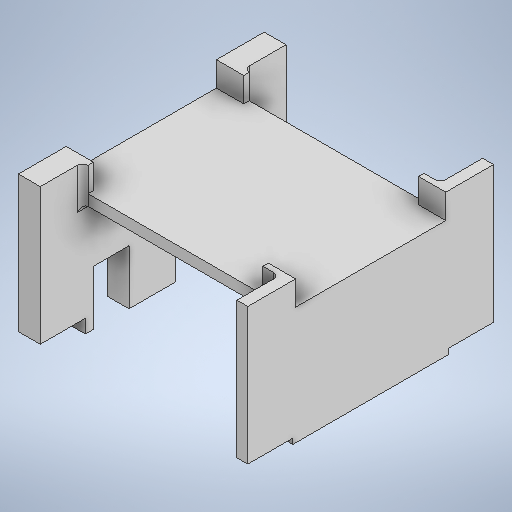
# Autodesk Inventor part: Breadboard_insert
Saved by Autodesk Inventor 2025.2 (Build 292293000, 293)
## iProperties
Created: 2025-09-19
Part Number: Breadboard_insert
Material: Generic
Document SubType Name: Modeling
Designer: TSO
Density: 1 g/cm^3
Appearance: Default
Author: TSO
Autodesk Inventor part; units mm, degrees
ref_plane "YZ Plane" through (0, 0, 0) normal (1, 0, 0) x (0, 1, 0)
ref_plane "XZ Plane" through (0, 0, 0) normal (0, 1, 0) x (-1, 0, 0)
ref_plane "XY Plane" through (0, 0, 0) normal (0, 0, 1) x (1, 0, 0)
sketch "Sketch1" plane through (0, 0, 0) normal (0, 1, 0) x (-1, 0, 0)
  line L0 (0, 0) -> (84, 0)
  line L1 (84, 0) -> (84, -90)
  line L2 (84, -90) -> (0, -90)
  line L3 (0, -90) -> (0, 0)
  line L4 (84, 0) -> (76, 0)
  line L5 (76, 0) -> (4, 0)
  line L6 (4, 0) -> (4, -15.5)
  line L7 (4, -15.5) -> (76, -15.5)
  line L8 (76, -15.5) -> (76, 0)
  line L9 (84, -45) -> (0, -45) construction
  line L10 (4, -90) -> (4, -74.5)
  line L11 (4, -74.5) -> (76, -74.5)
  line L12 (76, -74.5) -> (76, -90)
  point P0 (4, 0)
  point P1 (4, -90)
  dimension "d0" = 84
  dimension "d1" = 90
  dimension "d4" = 8
  dimension "d5" = 72
  dimension "d6" = 15.5
  constraints: 26 end point, 4 parallel, 4 symmetric about line, 2 horizontal, 2 midpoint, 2 perpendicular, 1 point on line
  measures "d0" distance of L1.end L2.end
  measures "d1" distance of L0.end L1.end
  measures "d4" distance of L0.end L4.end
  measures "d5" distance of L7.end L6.end
  measures "d6" distance of L6.end L5.end
extrude "Extrusion1" add sketch "Sketch1" along normal blind 4 contours L0 L6 L7 L8 L1 L2 L12 L11 L10 L3
sketch "Sketch2" plane through (0, 0, 0) normal (0, -1, 0) x (1, 0, 0)
  line L0 (-84, -90) -> (-84, 0) projected
  line L1 (-76, 0) -> (-76, -15.5) projected
  line L2 (-84, -90) -> (-76, -90)
  line L3 (-76, -90) -> (-76, 0)
  line L4 (-76, 0) -> (-84, 0)
  line L5 (-84, 0) -> (-84, -90)
  line L6 (0, -90) -> (0, 0)
  line L7 (0, 0) -> (0, -90) projected
  line L8 (-4, 0) -> (0, 0) projected
  line L9 (0, -90) -> (-4, -90)
  line L10 (-4, -90) -> (-4, 0)
  line L11 (-4, 0) -> (0, 0)
  line L12 (0, 0) -> (0, -90)
  dimension "d12" = 4
  constraints: 18 end point, 4 parallel, 2 horizontal, 2 perpendicular, 1 point on line
  measures "d12" distance of L10.end L11.end
extrude "Extrusion2" add sketch "Sketch2" along normal blind 37
sketch "Sketch3" plane through (0, -37, 0) normal (0, -1, 0) x (1, 0, 0)
  line L0 (-76, -74.5) -> (-76, -90) projected
  line L1 (-76, -74.5) -> (-76, -73.5)
  line L2 (-76, -15.5) -> (-76, -74.5) projected
  line L3 (-76, -73.5) -> (-84, -73.5)
  line L4 (-84, -73.5) -> (-84, -16.5)
  line L5 (-84, -16.5) -> (-76, -16.5)
  line L6 (-76, -16.5) -> (-76, -73.5)
  point P0 (0, 0)
  dimension "d17" = 1
  dimension "d18" = 8
  dimension "d19" = 57
  constraints: 10 end point, 2 parallel, 1 horizontal, 1 perpendicular, 1 point on line
  measures "d17" distance of L0.start L1.end
  measures "d18" distance of L4.end L5.end
  measures "d19" distance of L3.end L4.end
extrude "Extrusion3" add sketch "Sketch3" along normal blind 5
sketch "Sketch5" plane through (0, -37, 0) normal (0, -1, 0) x (1, 0, 0)
  line L0 (-4, -74.5) -> (-4, -73.5)
  line L1 (-4, -73.5) -> (-4, -73.5) construction
  line L2 (-4, 0) -> (-4, -90) projected
  line L3 (-4, -73.5) -> (0, -73.5)
  line L4 (0, -73.5) -> (0, -16.5)
  line L5 (0, -16.5) -> (-4, -16.5)
  line L6 (-4, -16.5) -> (-4, -73.5)
  point P0 (0, 0)
  dimension "d20" = 1
  dimension "d21" = 4
  dimension "d22" = 57
  constraints: 12 end point, 2 parallel, 2 perpendicular, 1 horizontal, 1 point on line, 1 vertical
  measures "d20" distance of L0.start L0.end
  measures "d21" distance of L5.end L4.end
  measures "d22" distance of L4.end L3.end
extrude "Extrusion4" add sketch "Sketch5" along normal blind 2
fillet "Fillet1" radius 2 6 edges at (-76, 2, -15.5) (-76, 0, -45) (-76, 2, -74.5) (-4, 2, -74.5) (-4, 0, -45) (-4, 2, -15.5)
sketch "Sketch6" plane through (0, 4, 0) normal (0, 1, 0) x (1, 0, 0)
  line L0 (-6, 74.5) -> (-74, 74.5) projected
  line L1 (-26.2554, 74.5) -> (0, 74.5) construction
  line L2 (0, 74.5) -> (-10, 74.5)
  line L3 (-10, 74.5) -> (-10, 72.5)
  line L4 (-10, 72.5) -> (0, 72.5)
  line L5 (0, 72.5) -> (0, 74.5)
  line L6 (-100.2554, 74.5) -> (-74, 74.5) construction
  line L7 (-84, 74.5) -> (-84, 72.5)
  line L8 (-84, 72.5) -> (-74, 72.5)
  line L9 (-74, 74.5) -> (-84, 74.5)
  line L10 (-74, 72.5) -> (-74, 74.5)
  line L11 (-26.2554, 17.5) -> (0, 17.5) construction
  line L12 (-10, 17.5) -> (-10, 15.5)
  line L13 (-10, 15.5) -> (0, 15.5)
  line L14 (0, 17.5) -> (-10, 17.5)
  line L15 (0, 15.5) -> (0, 17.5)
  line L16 (-100.2554, 17.5) -> (-74, 17.5) construction
  line L17 (-84, 17.5) -> (-84, 15.5)
  line L18 (-84, 15.5) -> (-74, 15.5)
  line L19 (-74, 17.5) -> (-84, 17.5)
  line L20 (-74, 15.5) -> (-74, 17.5)
  line L21 (-84, 0) -> (-76, 0) projected
  line L22 (-84, 0) -> (-76, 0)
  line L23 (-76, 0) -> (-76, 15.5)
  line L24 (-76, 15.5) -> (-84, 15.5)
  line L25 (-84, 15.5) -> (-84, 0)
  line L26 (-76, 76.5) -> (-76, 90) projected
  line L27 (-76, 90) -> (-84, 90)
  line L28 (-84, 90) -> (-84, 74.5)
  line L29 (-84, 74.5) -> (-76, 74.5)
  line L30 (-76, 74.5) -> (-76, 90)
  line L31 (-4, 90) -> (-4, 76.5) projected
  line L32 (-4, 90) -> (0, 90)
  line L33 (0, 90) -> (0, 74.5)
  line L34 (0, 74.5) -> (-4, 74.5)
  line L35 (-4, 74.5) -> (-4, 90)
  line L36 (-4, 0) -> (0, 0) projected
  line L37 (-4, 0) -> (0, 0)
  line L38 (0, 0) -> (0, 15.5)
  line L39 (0, 15.5) -> (-4, 15.5)
  line L40 (-4, 15.5) -> (-4, 0)
  dimension "d26" = 10
  dimension "d27" = 2
  dimension "d30" = 74
  dimension "d33" = 57
  constraints: 72 end point, 10 parallel, 7 horizontal, 5 perpendicular, 2 point on line, 1 collinear, 1 vertical, 29 other
  measures "d26" distance of L4.end L3.end
  measures "d27" distance of L3.end L2.end
  measures "d30" distance of L1.start L6.start
  measures "d33" distance of L1.start L11.start
extrude "Extrusion5" add sketch "Sketch6" along normal blind 9
fillet "Fillet2" radius 2 4 edges at (-76, 8.5, -15.5) (-4, 8.5, -15.5) (-4, 8.5, -74.5) (-76, 8.5, -74.5)
sketch "Sketch8" plane through (-84, -42, -73.5) normal (-1, 0, 0) x (0, 0, 1)
  line L0 (-16.5, 5) -> (-16.5, 55) projected
  line L1 (-16.5, 5) -> (8, 5)
  line L2 (0, 3) -> (57, 3) projected
  line L3 (-16.5, 5) -> (8, 5) construction
  line L4 (24, 5) -> (24, 20)
  line L5 (24, 20) -> (8, 20)
  line L6 (8, 20) -> (8, 5)
  line L7 (57, 0) -> (0, 0) projected
  line L8 (8, 5) -> (8, 0)
  line L9 (8, 0) -> (24, 0)
  line L10 (24, 0) -> (24, 5)
  line L11 (73.5, 5) -> (73.5, 55) projected
  line L12 (73.5, 5) -> (54, 5)
  line L13 (54, 5) -> (54, 20)
  line L14 (54, 20) -> (73.5, 20)
  line L15 (73.5, 20) -> (73.5, 5)
  line L16 (54, 20) -> (41, 20)
  line L17 (41, 20) -> (41, 0)
  line L18 (41, 0) -> (54, 0)
  line L19 (54, 0) -> (54, 20)
  point P0 (73.5, 42)
  dimension "d39" = 24.5
  dimension "d40" = 0
  dimension "d41" = 16
  dimension "d42" = 15
  dimension "d44" = 19.5
  dimension "d45" = 15
  dimension "d46" = 13
  constraints: 32 end point, 7 parallel, 3 horizontal, 2 perpendicular, 2 point on line, 1 collinear
  measures "d39" distance of L0.start L1.end
  measures "d40" distance between parallel lines of L1 L3
  measures "d41" distance of L5.end L4.end
  measures "d42" distance of L4.end L4.start
  measures "d44" distance of L13.end L14.end
  measures "d45" distance of L12.end L13.end
  measures "d46" distance of L18.end L17.end
extrude "Extrusion6" cut sketch "Sketch8" against normal up to surface (8 mm away) contours L8 L6 L5 L4 L10 L2 | L2 L10 L7 L8 | L17 L16 L13 L19 L2 | L2 L19 L7 L17
body "Solid1"
